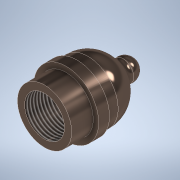
# Autodesk Inventor part: 3. 砲尾
Saved by Autodesk Inventor 2022 (Build 260153000, 153)
## iProperties
Created: 2023-05-12
Part Number: 3. 砲尾
Material: 一般
Document SubType Name: Modeling
Designer: USER
Density: 1 g/cm^3
Appearance: 砲銅 - 古董色拋光
Author: USER
Autodesk Inventor part; units mm, degrees
ref_plane "YZ Plane" through (0, 0, 0) normal (1, 0, 0) x (0, 1, 0)
ref_plane "XZ Plane" through (0, 0, 0) normal (0, 1, 0) x (-1, 0, 0)
ref_plane "XY Plane" through (0, 0, 0) normal (0, 0, 1) x (1, 0, 0)
sketch "草圖1" plane through (0, 0, 0) normal (1, 0, 0) x (0, 1, 0)
  arc A0 (0, -5) -> (0, 5) centre (0, 0) ccw
  line L0 (0, 27) -> (12.5, 27)
  line L1 (12.5, 27) -> (12.5, 37)
  line L2 (12.5, 37) -> (0, 37)
  line L3 (0, 27) -> (15, 27)
  line L4 (15, 27) -> (15, 22)
  line L5 (15, 22) -> (0, 22)
  line L6 (0, 22) -> (0, 27)
  arc A1 (0, 3) -> (0, 31) centre (0, 17) ccw
  line L7 (14, 22) -> (14, 17)
  line L8 (0, 37) -> (0, -5)
  point P0 (3.5993, 3.4706)
  dimension "d0" = 10
  dimension "d2" = 12.5
  dimension "d3" = 10
  dimension "d4" = 15
  dimension "d10" = 20
  dimension "d11" = 5
  dimension "d12" = 27
  constraints: 18 end point, 5 point on circle, 3 parallel, 2 centre point, 2 horizontal, 2 perpendicular, 2 vertical, 1 coincident, 1 point on line, 1 tangent
  measures "d0" diameter of A0
  measures "d2" distance of L2.end L1.end
  measures "d3" distance of L1.end L0.end
  measures "d4" distance of L4.end L5.end
  measures "d10" distance from line of A1.centre L2
  measures "d11" distance of L3.end L4.end
  measures "d12" distance of point (0, 0) L0.start
revolve "迴轉1" add sketch "草圖1" angle 360 about axis through (0, 0, 37) along (0, 0, -1)
fillet "圓角1" radius 4 1 edges at (0, -3.5993, 3.4706)
sketch "草圖2" plane through (0, 0, 37) normal (0, 0, 1) x (1, 0, 0)
  point P0 (0, 0)
  point P1 (0, 0)
  constraints: 1 coincident
hole "孔1" at (0, 0, 37) direction (0, 0, -1) diameter 18 depth 25 tip angle 118
sketch "草圖3" plane through (0, 0, 37) normal (0, 0, 1) x (1, 0, 0)
  point P0 (0, 0)
  point P1 (0, 0)
  constraints: 1 coincident
hole "孔2" at (0, 0, 37) direction (0, 0, -1) diameter 18.376 depth 20 thread size "M20x1.5" class "6H" standard "ISO Metric profile"
